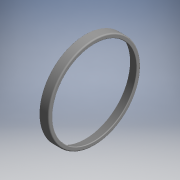
# Autodesk Inventor part: T4DB 170_or
Saved by Autodesk Inventor 2017.3 (Build 213256000, 256)
## iProperties
Part Number: T4DB 170_or
Material: Generic
Catalog Web Link: www.cadenas.de
Description: BT1_001_101_outer_ring-Tapered roller bearings, single row
Vendor: SKF
Document SubType Name: Modeling
Designer: partserver
Manufacturer: SKF
Mass: 110.349 g
Surface Area: 406.097 cm^2
Volume: 110.349 cm^3
Density: 1 g/cm^3
Appearance: PSOLRGB-175-175-175
Category: PARTsolutions
Company: SKF
Title: T4DB 170_or
Author: Cadenas PARTsolutions
Comments: Tapered roller bearings, single row
PSOL_IDENT_0: {$CADENAS_DATA\23d-libs\skf\bearings_units_and_housings\roller_bearings\tapered_roller_bearings\tape
PSOL_IDENT_1: red_roller_bearings_single_row\parts\bt1_001_101_or.prj},180 {VTYP=3D},{NB=T4DB 170_or},{LINA=T4DB 1
PSOL_IDENT_2: 70_or},{NN=BT1_001_101_outer_ring},{DATE=23.12.2020 07:01:44},{GEOMDATE=04.11.2020 10:41:00},{VERSIO
PSOL_IDENT_3: N=},{LINEID=4320},{WBVAR=},{WBNUMERIC=}  {NB=T4DB 170_or},{LINA=T4DB 170_or},{KT=DUMMY},{DESIGNATION=
PSOL_IDENT_4: T4DB 170},{DD=170.000},{D=230.000},{T=32.000},{DD1=197.5000},{D1=MIN},{ALPHA=17.100},{RANGLE=2.500},
PSOL_IDENT_5: {IRA=14.600},{B=30.000},{C=23.000},{C1=MIN},{R12=3.0},{R34=3.0},{AA=44.29541},{PITCH=200.033},{DW=16
PSOL_IDENT_6: .450},{LW=21.500},{DDAMAX=182},{DDAMIN=184.5},{DAMIN=215},{DAMAX=216.0},{DBMIN=223},{CA=6},{CB=9.0},
PSOL_IDENT_7: {RA=3.0},{RB=3.0},{LOAD1=307.000},{LOAD2=440.000},{LOAD3=43.000},{SPEED1=2000},{SPEED2=2600},{EE=0.4
PSOL_IDENT_8: 6},{Y=1.30},{Y0=0.7},{Y1=0},{X1=1},{X2=0.4},{X0=0.5},{Z=37},{II=1},{R1=0.00000231},{R2=10.9},{S1=0.0
PSOL_IDENT_9: 19},{S2=2},{KZ=6},{KL=0.7},{BF=2},{MASS=3.439},{DESIGN=trb1},{HELP=0.000},{PPATH=parts/bt1_001_101_a
PSOL_IDENT_10: smtpl.prj},{SUPPRESS=N},{A4=200000},{A15=350000},{BEARING=T4DB 170},{A8=300000},{POPULAR=}
NB: T4DB 170_or
NN: BT1_001_101_outer_ring
NT: Tapered roller bearings, single row
NBSYN: $DESIGNATION._or
LINA: T4DB 170_or
CATALOG: SKF
DESIGNATION: T4DB 170
DD: 170
D: 230
T: 32
DD1: 197.5
D1: 0
ALPHA: 17.1
RANGLE: 2.5
IRA: 14.6
B: 30
C: 23
C1: 0
R12: 3
R34: 3
AA: 44.29541
PITCH: 200.033
DW: 16.45
LW: 21.5
DDAMAX: 182
DDAMIN: 184.5
DAMIN: 215
DAMAX: 216
DBMIN: 223
CA: 6
CB: 9
RA: 3
RB: 3
LOAD1: 307
LOAD2: 440
LOAD3: 43
SPEED1: 2000
SPEED2: 2600
EE: 0.46
Y: 1.3
Y0: 0.7
Y1: 0
X1: 1
X2: 0.4
X0: 0.5
Z: 37
II: 1
R1: 0.00000231
R2: 10.9
S1: 0.019
S2: 2
KZ: 6
KL: 0.7
BF: 2
MASS: 3.439
PPATH: parts/bt1_001_101_asmtpl.prj
SUPPRESS: N
A4: 200000
A15: 350000
BEARING: T4DB 170
A8: 300000
SUPPLIER: SKF
ARTICLENO: T4DB 170_or
BOMINFO: T4DB 170_or
CREATOR: CADENAS GmbH
Autodesk Inventor part; units mm, degrees
sketch "Sketch_1" plane through (0, 0, 0) normal (0, 0, 1) x (1, 0, 0)
  line L0 (23, 0) -> (-23, 0)
  arc A0 (0, 106.4915) -> (1.9411, 105.0578) centre (1.5, 106.4915) ccw
  line L1 (1.9411, 105.0578) -> (23, 111.5364)
  line L2 (23, 111.5364) -> (23, 114)
  arc A1 (23, 114) -> (22, 115) centre (22, 114) ccw
  line L3 (22, 115) -> (3, 115)
  arc A2 (3, 115) -> (0, 112) centre (3, 112) ccw
  line L4 (0, 112) -> (0, 106.4915)
  constraints: 10 end point, 6 point on circle, 3 centre point
revolve "Revolution1" add sketch "Sketch_1" angle 360 about axis through (23, 0, 0) along (1, 0, 0)
ref_plane "outer_ring_XY" through (0, 0, 0) normal (0, 0, 1) x (1, 0, 0)
ref_plane "outer_ring_YZ" through (0, 0, 0) normal (1, 0, 0) x (0, 1, 0)
ref_plane "outer_ring_ZX" through (0, 0, 0) normal (0, 1, 0) x (0, 0, 1)
body "Solid1"
